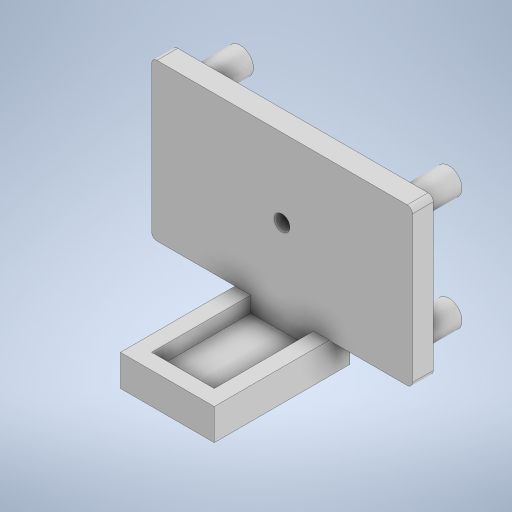
# Autodesk Inventor part: reward v06
Saved by Autodesk Inventor 2023 (Build 270158000, 158)
## iProperties
Created: 2022-07-15
Part Number: reward v06
Material: Generic
Document SubType Name: Modeling
Designer: ledap
Density: 1 g/cm^3
Appearance: Default
Author: ledap
Autodesk Inventor part; units mm, degrees
ref_plane "YZ Plane" through (0, 0, 0) normal (1, 0, 0) x (0, 1, 0)
ref_plane "XZ Plane" through (0, 0, 0) normal (0, 1, 0) x (-1, 0, 0)
ref_plane "XY Plane" through (0, 0, 0) normal (0, 0, 1) x (1, 0, 0)
sketch "Sketch1" plane through (0, 0, 0) normal (0, 0, 1) x (1, 0, 0)
  line L0 (25, 15) -> (-25, 15)
  line L1 (-25, 15) -> (-25, -15)
  line L2 (-25, -15) -> (25, -15)
  line L3 (25, -15) -> (25, 15)
  line L4 (25, 15) -> (-25, -15) construction
  line L5 (-25, 15) -> (25, -15) construction
  point P0 (0, 0)
  dimension "d0" = 50
  dimension "d1" = 30
  constraints: 12 end point, 2 midpoint, 2 parallel, 1 horizontal, 1 perpendicular
  measures "d0" distance of L2.end L1.end
  measures "d1" distance of L1.end L0.end
extrude "Extrusion1" add sketch "Sketch1" along normal blind 4
fillet "Fillet1" radius 1 1 edges at (25, 15, 2)
fillet "Fillet2" radius 1 3 edges at (-25, 15, 2) (25, -15, 2) (-25, -15, 2)
sketch "Sketch4" plane through (0, 0, 4) normal (0, 0, 1) x (1, 0, 0)
  circle A0 centre (0, 0) radius 1.5
  dimension "d19" = 3
  constraints: 1 centre point, 1 coincident
  measures "d19" diameter of A0
hole "Hole2" at (0, 0, 4) direction (0, 0, -1) diameter 3 end through all both
sketch "Sketch6" plane through (0, 0, 4) normal (0, 0, 1) x (1, 0, 0)
  circle A0 centre (-20, 11) radius 2.5
  circle A1 centre (20, 11) radius 2.5
  circle A2 centre (-20, -11) radius 2.5
  circle A3 centre (20, -11) radius 2.5
  line L0 (25, -14) -> (25, 14) projected
  line L1 (-25, 14) -> (-25, -14) projected
  line L2 (24, 15) -> (-24, 15) projected
  line L3 (-24, -15) -> (24, -15) projected
  point P0 (0, 0)
  dimension "d27" = 5
  dimension "d28" = 5
  dimension "d29" = 5
  dimension "d30" = 5
  dimension "d38" = 5
  dimension "d39" = 5
  dimension "d40" = 5
  dimension "d41" = 5
  dimension "d42" = 4
  dimension "d43" = 4
  dimension "d44" = 4
  dimension "d45" = 4
  constraints: 4 centre point
  measures "d27" diameter of A0
  measures "d28" diameter of A1
  measures "d29" diameter of A2
  measures "d30" diameter of A3
  measures "d38" distance from line of L0 A1.centre
  measures "d39" distance from line of L0 A3.centre
  measures "d40" distance from line of L1 A0.centre
  measures "d41" distance from line of L1 A2.centre
  measures "d42" distance from line of A0.centre L2
  measures "d43" distance from line of L2 A1.centre
  measures "d44" distance from line of L3 A2.centre
  measures "d45" distance from line of L3 A3.centre
sketch "Sketch18" plane through (0, 0, 0) normal (0, 0, -1) x (-1, 0, 0)
  point P0 (0, 0)
extrude "Extrusion10" add sketch "Sketch6" against normal blind 12
sketch "Sketch19" plane through (0, 0, 0) normal (0, 0, -1) x (-1, 0, 0)
  line L0 (24, -15) -> (-24, -15) projected
  line L1 (-9, -15) -> (9, -15)
  line L2 (9, -15) -> (9, -21)
  line L3 (9, -21) -> (-9, -21)
  line L4 (-9, -21) -> (-9, -15)
  point P0 (0, 0)
  dimension "d84" = 18
  dimension "d85" = 6
  constraints: 8 end point, 2 parallel, 1 horizontal, 1 perpendicular, 1 point on line
  measures "d84" distance of L2.end L3.end
  measures "d85" distance of L1.end L2.end
extrude "Extrusion11" add sketch "Sketch19" against normal blind 26
sketch "Sketch20" plane through (-9, -15, 4) normal (0, 1, 0) x (1, 0, 0)
  point P0 (9, 4)
sketch "Sketch21" plane through (-9, -15, 4) normal (0, 1, 0) x (1, 0, 0)
  line L0 (33, 0) -> (-15, 0) projected
  line L1 (3, 0) -> (15, 0)
  line L2 (15, 0) -> (15, -19)
  line L3 (15, -19) -> (3, -19)
  line L4 (3, -19) -> (3, 0)
  point P0 (9, 4)
  dimension "d88" = 12
  dimension "d89" = 19
  constraints: 8 end point, 2 parallel, 1 horizontal, 1 perpendicular, 1 point on line
  measures "d88" distance of L2.end L3.end
  measures "d89" distance of L1.end L2.end
extrude "Extrusion12" cut sketch "Sketch21" against normal blind 3
body "Solid1"
